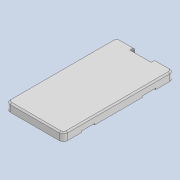
# Autodesk Inventor part: scatola_v2_sopra
Saved by Autodesk Inventor 2022 (Build 260153000, 153)
## iProperties
Created: 2025-09-23
Part Number: scatola_v2_sopra
Material: Generic
Document SubType Name: Modeling
Designer: 1234
Density: 1 g/cm^3
Appearance: Default
Author: 1234
Autodesk Inventor part; units mm, degrees
ref_plane "YZ Plane" through (0, 0, 0) normal (1, 0, 0) x (0, 1, 0)
ref_plane "XZ Plane" through (0, 0, 0) normal (0, 1, 0) x (-1, 0, 0)
ref_plane "XY Plane" through (0, 0, 0) normal (0, 0, 1) x (1, 0, 0)
sketch "Sketch1" plane through (0, 0, 0) normal (0, 1, 0) x (-1, 0, 0)
  line L0 (0, 0) -> (35.4, 0)
  line L1 (35.4, 0) -> (35.4, 75.4)
  line L2 (35.4, 75.4) -> (0, 75.4)
  line L3 (0, 75.4) -> (0, 0)
  line L4 (39.2, -3.8) -> (-3.8, -3.8)
  line L5 (-3.8, -3.8) -> (-3.8, 79.2)
  line L6 (-3.8, 79.2) -> (39.2, 79.2)
  line L7 (39.2, 79.2) -> (39.2, -3.8)
  line L8 (39.2, 37.7) -> (49.7975, 37.7) construction
  line L9 (17.7, 79.2) -> (17.7, 95.7522) construction
  line L10 (24.7, 75.4) -> (21.7, 75.4)
  line L11 (21.7, 75.4) -> (21.7, 68.4)
  line L12 (21.7, 68.4) -> (24.7, 68.4)
  line L13 (24.7, 68.4) -> (24.7, 75.4)
  line L14 (13.7, 75.4) -> (10.7, 75.4)
  line L15 (10.7, 75.4) -> (10.7, 68.4)
  line L16 (10.7, 68.4) -> (13.7, 68.4)
  line L17 (13.7, 68.4) -> (13.7, 75.4)
  line L18 (0.2, 75.2) -> (35.2, 75.2)
  line L19 (35.2, 75.2) -> (35.2, 0.2)
  line L20 (35.2, 0.2) -> (0.2, 0.2)
  line L21 (0.2, 0.2) -> (0.2, 75.2)
  point P0 (21.7, 75.4)
  point P1 (10.7, 75.4)
  dimension "d43" = 4
  dimension "d44" = 4
  dimension "d45" = 7
  dimension "d46" = 3
  dimension "d47" = 3
  dimension "d74" = 0.2
  dimension "d75" = 75
  dimension "d76" = 35
  dimension "d77" = 4
  constraints: 44 end point, 10 parallel, 5 perpendicular, 4 horizontal, 3 point on line, 2 midpoint, 1 vertical, 6 other
  measures "d43" distance between parallel lines of L9 L17
  measures "d44" distance between parallel lines of L9 L11
  measures "d45" distance of L12.end L10.start
  measures "d46" distance of L11.end L12.end
  measures "d47" distance of L15.end L16.end
  measures "d74" distance between parallel lines of L2 L18
  measures "d75" distance of L18.end L19.end
  measures "d76" distance of L18.start L18.end
  measures "d77" distance between parallel lines of L20 L4
extrude "Extrusion1" add sketch "Sketch1" along normal blind 6 contours L3 L2 L15 L18 L21 L20 L19 L13 L1 L0 | L2 L17 L18 L15 | L13 L18 L11 L2 | L2 L11 L18 L17 | L18 L17 L16 L15 | L15 L16 L17 L18 L11 L12 L13 L19 L20 L21 | L13 L12 L11 L18 | L4 L5 L6 L7
extrude "Extrusion2" cut sketch "Sketch1" along normal blind 5 contours L3 L2 L15 L18 L21 L20 L19 L13 L1 L0 | L2 L11 L18 L17 | L15 L16 L17 L18 L11 L12 L13 L19 L20 L21
sketch "Sketch3" plane through (5, 0, -3.8) normal (0, 0, -1) x (-1, 0, 0)
  line L0 (22.7, 10) -> (22.7, 15.0736) construction
  line L1 (29.7, 8) -> (15.7, 8)
  line L2 (14.7, 7) -> (14.7, 0)
  line L3 (30.7, 0) -> (30.7, 7)
  arc A0 (30.7, 7) -> (29.7, 8) centre (29.7, 7) ccw
  arc A1 (15.7, 8) -> (14.7, 7) centre (15.7, 7) ccw
  line L4 (30.7, 0) -> (14.7, 0)
  line L5 (1.2, 0) -> (44.2, 0) projected
  line L6 (44.2, 0) -> (1.2, 0) projected
  line L7 (17.7, 0) -> (17.7, 4.1)
  line L8 (18.7, 5.1) -> (26.7, 5.1)
  line L9 (27.7, 4.1) -> (27.7, 0)
  arc A2 (18.7, 5.1) -> (17.7, 4.1) centre (18.7, 4.1) ccw
  arc A3 (27.7, 4.1) -> (26.7, 5.1) centre (26.7, 4.1) ccw
  line L10 (1.2, 0) -> (1.2, 6) projected
  line L11 (44.2, 0) -> (44.2, 6) projected
  point P0 (30.5, 8)
  point P1 (14.5, 8)
  point P2 (17.7, 0)
  dimension "d15" = 8
  dimension "d16" = 8
  dimension "d19" = 1
  dimension "d27" = 5.1
  dimension "d28" = 5
  dimension "d29" = 5
  dimension "d30" = 1
  dimension "d33" = 21.5
  dimension "d34" = 43
  dimension "d35" = 8
  constraints: 16 end point, 8 point on circle, 8 tangent, 4 centre point, 4 vertical, 2 equal radius, 2 perpendicular, 2 point on line, 1 collinear, 1 horizontal, 1 parallel
  measures "d15" distance between parallel lines of L0 L3
  measures "d16" distance between parallel lines of L2 L0
  measures "d19" radius of A0
  measures "d27" distance between parallel lines of L5 L8
  measures "d28" distance between parallel lines of L0 L9
  measures "d29" distance between parallel lines of L0 L7
  measures "d30" radius of A2
  measures "d33" distance between parallel lines of L10 L0
  measures "d34" distance between parallel lines of L10 L11
  measures "d35" distance between parallel lines of L1 L4
extrude "Extrusion3" cut sketch "Sketch3" against normal up to surface (3.8 mm away) contours L4 L7 A2 L8 A3 L9
extrude "Extrusion4" cut sketch "Sketch3" against normal blind 3.5 contours A0 L3 L4 L9 A3 L8 A2 L7 L2 A1 L1
fillet "Fillet1" radius 3 4 edges at (3.8, 3, -3.8) (-39.2, 3, -3.8) (3.8, 3, 79.2) (-39.2, 3, 79.2)
chamfer "Chamfer3" distance 1 angle 45 9 edges at (-4.45, 6, -3.8) (-30.95, 6, -3.8) (-38.3213, 6, -2.9213) (-39.2, 6, 37.7) (-38.3213, 6, 78.3213) (-17.7, 6, 79.2) (2.9213, 6, 78.3213) (3.8, 6, 37.7) (2.9213, 6, -2.9213)
fillet "Fillet2" radius 1 4 edges at (-24.7, 2.5, 75.4) (-21.7, 2.5, 75.4) (-13.7, 2.5, 75.4) (-10.7, 2.5, 75.4)
chamfer "Chamfer5" distance 1 angle 45 4 edges at (-24.7, 2.5, 68.4) (-21.7, 2.5, 68.4) (-13.7, 2.5, 68.4) (-10.7, 2.5, 68.4)
ref_plane "Work Plane2" through (0.8, 0, 67.7) normal (0, 0, -1) x (-1, 0, 0)
ref_plane "Work Plane1" through (0.8, 0, 37.7) normal (0, 0, -1) x (-1, 0, 0)
ref_plane "Work Plane3" through (-17.7, 0, 76.2) normal (1, 0, 0) x (0, 0, -1)
ref_plane "Work Plane4" through (0.8, 0, 65.7) normal (0, 0, -1) x (-1, 0, 0)
sketch "Sketch4" plane through (0.8, 0, 37.7) normal (0, 0, -1) x (-1, 0, 0)
  line L0 (36.2, 0) -> (36.2, 5) projected
  line L1 (36.2, 0) -> (37.8, 0) construction
  line L2 (40, 0) -> (36.2, 0) projected
  line L3 (37.8, 0) -> (37.8, 5) construction
  line L4 (38.15, 4.65) -> (38.15, 3.9) construction
  line L5 (37.8, 5) -> (36.2, 5) construction
  line L6 (37.8, 5) -> (38.15, 4.65) construction
  line L7 (38.15, 3.9) -> (37.8, 3.55) construction
  line L8 (38.4, 0) -> (37.97, 3)
  line L9 (37.97, 3) -> (37.97, 3.72)
  line L10 (37.97, 3.72) -> (38.25, 4)
  line L11 (38.25, 4) -> (38.25, 5.1)
  line L12 (36.2, 0) -> (0.8, 0) projected
  line L13 (38.4, 0) -> (36.2, 0)
  line L14 (36.2, 0) -> (36.2, 5)
  line L15 (38.25, 5.1) -> (36.2, 5.1)
  line L16 (36.2, 5.1) -> (36.2, 5)
  line L17 (37, 0) -> (37, 5) projected
  line L18 (36.2, 5.1) -> (36.1, 5)
  line L19 (36.2, 5) -> (26.5, 5) projected
  line L20 (36.2, 5) -> (36.1, 5)
  dimension "d53" = 1.6
  dimension "d54" = 5
  dimension "d55" = 0.35
  dimension "d58" = 45
  dimension "d59" = 45
  dimension "d60" = 1.1
  dimension "d61" = 0.17
  dimension "d62" = 0.6
  dimension "d63" = 3
  dimension "d64" = 0.1
  dimension "d83" = 135
  dimension "d84" = 0.1
  constraints: 33 end point, 7 point on line, 4 vertical, 3 horizontal, 2 perpendicular, 1 other
  measures "d53" distance of L0.start L1.end
  measures "d54" distance of L1.end L3.end
  measures "d55" distance between parallel lines of L3 L4
  measures "d58" angle of L3 L6
  measures "d59" angle of L3 L7
  measures "d60" distance from line of L5 L4.end
  measures "d61" distance between parallel lines of L3 L9
  measures "d62" distance from line of L3 L8.start
  measures "d63" distance from line of L1 L8.end
  measures "d64" distance between parallel lines of L4 L11
  measures "d83" angle of L16 L18
  measures "d84" distance between parallel lines of L19 L15
sketch "Sketch5" plane through (0.8, 0, 67.7) normal (0, 0, -1) x (-1, 0, 0)
  line L0 (40, 5) -> (40, 0) projected
  line L1 (40, 1) -> (39, 0)
  line L2 (40, 0) -> (37, 0) projected
  line L3 (40, 1) -> (40, 0)
  line L4 (39, 0) -> (40, 0)
  point P0 (0.8, 0)
  dimension "d65" = 45
  dimension "d66" = 1
  constraints: 6 end point, 2 point on line, 1 collinear, 1 vertical
  measures "d65" angle of L2 L1
  measures "d66" distance from line of L1.end L0
extrude "Extrusion5" cut sketch "Sketch5" along normal blind 10 from surface at 2
extrude "Extrusion6" cut sketch "Sketch4" against normal blind 33
mirror "Mirror1" about plane through (0.8, 0, 37.7) normal (0, 0, -1) of "Extrusion6", "Extrusion5"
mirror "Mirror2" about plane through (-17.7, 0, 76.2) normal (1, 0, 0) of "Extrusion6", "Extrusion5", "Mirror1"
extrude "Extrusion7" cut sketch "Sketch1" along normal blind 0.1 contours L3 L2 L15 L18 L21 L20 L19 L13 L1 L0 | L2 L17 L18 L15 | L13 L18 L11 L2 | L2 L11 L18 L17 | L18 L17 L16 L15 | L15 L16 L17 L18 L11 L12 L13 L19 L20 L21 | L13 L12 L11 L18
equation "\"d43\" = d44"
equation "\"d47\" = d46"
equation "\"d16\" = d15"
equation "\"d29\" = d28"
equation "\"d33\" = 0.5 * d34"
body "Solid1"
